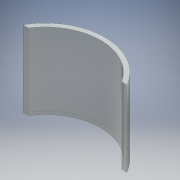
# Autodesk Inventor part: outsideCover2
Saved by Autodesk Inventor 2016 (Build 200138000, 138)
## iProperties
Created: 2016-11-11
Part Number: outsideCover2
Material: ガラス
Document SubType Name: Modeling
Designer: Daisuke
Density: 2.18 g/cm^3
Appearance: クリア
Author: Daisuke
Autodesk Inventor part; units mm, degrees
ref_plane "YZ Plane" through (0, 0, 0) normal (1, 0, 0) x (0, 1, 0)
ref_plane "XZ Plane" through (0, 0, 0) normal (0, 1, 0) x (-1, 0, 0)
ref_plane "XY Plane" through (0, 0, 0) normal (0, 0, 1) x (1, 0, 0)
sketch "スケッチ2" plane through (0, 0, 0) normal (0, 0, 1) x (1, 0, 0)
  line L0 (0, 0) -> (47.6314, 27.5) construction
  line L1 (0, 0) -> (55, 0) construction
  line L2 (0, 0) -> (-47.6314, 27.5) construction
  line L3 (0, 0) -> (55, 0) construction
  line L4 (0, 0) -> (47.6314, -27.5) construction
  line L5 (0, 0) -> (55, 0) construction
  line L6 (0, 0) -> (-47.6314, -27.5) construction
  line L7 (0, 0) -> (55, 0) construction
  arc A0 (42.9506, -27.5) -> (44.1673, -25.5) centre (0, 0) ccw
  line L8 (-47.6314, 27.5) -> (-42.9506, 27.5)
  line L9 (42.9506, 27.5) -> (47.6314, 27.5)
  arc A1 (47.6314, 27.5) -> (-47.6314, 27.5) centre (0, 0) ccw
  arc A2 (42.9506, 27.5) -> (-42.9506, 27.5) centre (0, 0) ccw
  arc A3 (42.9506, -27.5) -> (44.1673, -25.5) centre (0, 0) ccw
  dimension "d8" = 30
  dimension "d9" = 150
  dimension "d10" = 30
  dimension "d11" = 150
  dimension "d13" = 51
  constraints: 20 end point, 8 point on circle, 4 centre point, 4 coincident, 4 equal length, 4 horizontal, 1 point on line
  measures "d8" angle of L1 L0
  measures "d9" angle of L3 L2
  measures "d10" angle of L4 L5
  measures "d11" angle of L6 L7
  measures "d13" radius of A0
extrude "押し出し2" add sketch "スケッチ2" along normal blind 70
